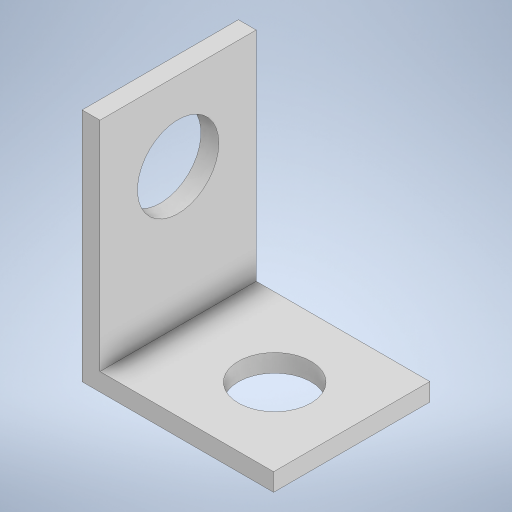
# Autodesk Inventor part: 615Bracket
Saved by Autodesk Inventor 2023.5 (Build 275446020, 446B)
## iProperties
Created: 2026-07-21
Part Number: 615Bracket
Material: Generic
Document SubType Name: Modeling
Designer: User
Density: 1 g/cm^3
Appearance: Default
Author: User
Autodesk Inventor part; units mm, degrees
ref_plane "YZ Plane" through (0, 0, 0) normal (1, 0, 0) x (0, 1, 0)
ref_plane "XZ Plane" through (0, 0, 0) normal (0, 1, 0) x (-1, 0, 0)
ref_plane "XY Plane" through (0, 0, 0) normal (0, 0, 1) x (1, 0, 0)
sketch "Sketch1" plane through (0, 0, 0) normal (0, 0, 1) x (1, 0, 0)
  line L0 (0, 0) -> (7.89, 0)
  line L1 (7.89, 0) -> (7.89, -0.81)
  line L2 (7.89, -0.81) -> (-0.81, -0.81)
  line L3 (-0.81, -0.81) -> (-0.81, 9.89)
  line L4 (-0.81, 9.89) -> (0, 9.89)
  line L5 (0, 9.89) -> (0, 0)
  dimension "d0" = 7.89
  dimension "d1" = 0.81
  dimension "d2" = 8.7
  dimension "d3" = 10.7
  constraints: 12 end point, 5 perpendicular, 1 horizontal
  measures "d0" distance of L0.start L0.end
  measures "d1" distance of L0.end L1.end
  measures "d2" distance of L1.end L2.end
  measures "d3" distance of L2.end L3.end
extrude "Extrusion1" add sketch "Sketch1" against normal blind 7.1
sketch "Sketch2" plane through (0, 0, 0) normal (0, 1, 0) x (1, 0, 0)
  line L0 (0, 0) -> (-0.81, 0) projected
  line L1 (-0.81, 7.1) -> (0, 7.1) projected
  line L2 (-0.81, 0) -> (-0.81, 7.1)
  line L3 (-0.81, 0) -> (-0.81, 7.1) projected
  line L4 (-0.81, 3.55) -> (4.39, 3.55)
  circle A0 centre (4.39, 3.55) radius 1.65
  dimension "d6" = 5.2
  dimension "d7" = 3.3
  constraints: 4 end point, 1 centre point, 1 coincident, 1 horizontal, 1 midpoint, 1 vertical
  measures "d6" distance of L4.start L4.end
  measures "d7" diameter of A0
extrude "Extrusion2" cut sketch "Sketch2" against normal blind 7.1
sketch "Sketch3" plane through (0, 0, 0) normal (1, 0, 0) x (0, 0, -1)
  line L0 (0, -0.81) -> (7.1, -0.81) projected
  line L1 (3.55, -0.81) -> (3.55, 6.29)
  circle A0 centre (3.55, 6.29) radius 1.85
  point P0 (0, 0)
  dimension "d10" = 7.1
  dimension "d11" = 3.7
  constraints: 2 end point, 1 centre point, 1 coincident, 1 midpoint, 1 vertical
  measures "d10" distance of L1.start L1.end
  measures "d11" diameter of A0
extrude "Extrusion3" cut sketch "Sketch3" against normal blind 7.1
body "Solid1"
